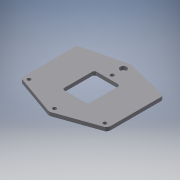
# Autodesk Inventor part: Corpo_Suporte_4_Cabos_Modelo2
Saved by Autodesk Inventor 2018 (Build 220112000, 112)
## iProperties
Created: 2021-08-02
Part Number: Corpo_Suporte_4_Cabos_Modelo2
Material: Generic
Document SubType Name: Modeling
Designer: L08619
Density: 1 g/cm^3
Appearance: Default
Author: L08619
Autodesk Inventor part; units mm, degrees
ref_plane "YZ Plane" through (0, 0, 0) normal (1, 0, 0) x (0, 1, 0)
ref_plane "XZ Plane" through (0, 0, 0) normal (0, 1, 0) x (-1, 0, 0)
ref_plane "XY Plane" through (0, 0, 0) normal (0, 0, 1) x (1, 0, 0)
sketch "Sketch1" plane through (0, 0, 0) normal (0, 0, 1) x (1, 0, 0)
  circle A0 centre (0, 0) radius 20
  circle A1 centre (-235, -350) radius 11
  circle A2 centre (235, -350) radius 11
  arc A3 (257.6264, -370.5094) -> (260.9808, -323.1206) centre (233.6625, -345) ccw
  circle A4 centre (0.0008, -70) radius 11
  line L0 (70, -100) -> (-70, -100)
  line L1 (-80, -110) -> (-80, -290)
  line L2 (-70, -300) -> (70, -300)
  line L3 (80, -290) -> (80, -110)
  line L4 (80, -100) -> (-80, -300) construction
  line L5 (-80, -100) -> (80, -300) construction
  line L6 (0, 64.9697) -> (0, -492.5476)
  arc A5 (-260.9808, -323.1206) -> (-257.6264, -370.5094) centre (-233.6625, -345) ccw
  line L7 (-80, -110) -> (-70, -100)
  line L8 (80, -110) -> (70, -100)
  line L9 (70, -300) -> (80, -290)
  line L10 (-70, -300) -> (-80, -290)
  arc A6 (20, 40.3113) -> (-20, 40.3113) centre (0, 0) ccw
  circle A7 centre (0, -427.5724) radius 11
  line L11 (-257.6264, -370.5094) -> (-11, -457.5724)
  arc A8 (-11, -457.5724) -> (11, -457.5724) centre (0, -426.4123) ccw
  line L12 (257.6264, -370.5094) -> (11, -457.5724)
  line L13 (-11, -457.5724) -> (11, -457.5724) construction
  line L14 (268.5751, -347.4713) -> (268.5751, -36.5544)
  line L15 (246, -14.5226) -> (20, 40.3113)
  line L16 (-268.5751, -347.4713) -> (-268.5751, -36.5544)
  line L17 (-246, -14.5226) -> (-20, 40.3113)
  line L18 (-268.5751, -36.5544) -> (-268.5751, -20) construction
  line L19 (-268.5751, -20) -> (-246, -14.5226) construction
  spline S0 degree 2 poles (-268.5751, -36.5544) (-268.5751, -20) (-246, -14.5226) knots 1 1 1 2 2 2
  line L20 (268.5751, -36.5544) -> (268.5751, -20) construction
  line L21 (268.5751, -20) -> (246, -14.5226) construction
  spline S1 degree 2 poles (268.5751, -36.5544) (268.5751, -20) (246, -14.5226) knots 1 1 1 2 2 2
  point P0 (0, -200)
  point P1 (0, -200)
  dimension "d0" = 40
  dimension "d3" = 22
  dimension "d4" = 22
  dimension "d9" = 35
  dimension "d33" = 22
  dimension "d35" = 160
  dimension "d36" = 200
  dimension "d37" = 70
  dimension "d38" = 30
  dimension "d39" = 10
  dimension "d40" = 10
  dimension "d41" = 10
  dimension "d42" = 10
  dimension "d43" = 10
  dimension "d44" = 10
  dimension "d45" = 10
  dimension "d46" = 10
  dimension "d47" = 45
  dimension "d50" = 22
  dimension "d51" = 30
  constraints: 36 end point, 10 point on circle, 9 centre point, 9 point on line, 4 symmetric about line, 3 midpoint, 2 coincident, 2 vertical, 1 collinear, 1 horizontal, 1 tangent, 6 other
  measures "d0" diameter of A0
  measures "d3" diameter of A1
  measures "d4" diameter of A2
  measures "d9" radius of A3
  measures "d33" diameter of A4
  measures "d35" distance of L4.start L5.start
  measures "d36" distance of L5.start L4.end
  measures "d37" distance of A4.centre A0.centre
  measures "d38" distance from line of L0 A4.centre
  measures "d39" distance of L1.start L5.start
  measures "d40" distance of L0.end L5.start
  measures "d41" distance of L3.end L4.start
  measures "d42" distance of L0.start L4.start
  measures "d43" distance of L2.end L5.end
  measures "d44" distance of L3.start L5.end
  measures "d45" distance of L2.start L4.end
  measures "d46" distance of L1.end L4.end
  measures "d47" radius of A6
  measures "d50" diameter of A7
  measures "d51" distance from line of A7.centre L13
extrude "Extrusion3" add sketch "Sketch1" along normal mid plane 22.22 contours A0 L6 A6 L15 S1 L14 A3 L12 A8 A7 L2 L9 L3 L8 L0 A4 | A0 L6 A4 L0 L7 L1 L10 L2 A7 A8 L11 A5 L16 S0 L17 A6
equation "\"d40\" = d39"
equation "\"d42\" = d41"
equation "\"d43\" = d41"
equation "\"d44\" = d43"
equation "\"d45\" = d41"
equation "\"d46\" = d45"
body "Solid3"
